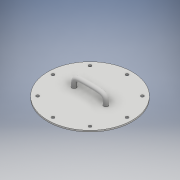
# Autodesk Inventor part: 人孔法兰
Saved by Autodesk Inventor 2018.2 (Build 222227000, 227)
## iProperties
Created: 2018-07-04
Part Number: 人孔法兰
Material: 常规
Document SubType Name: Modeling
Designer: Administrator
Density: 1 g/cm^3
Appearance: 默认
Author: Administrator
Autodesk Inventor part; units mm, degrees
ref_plane "YZ Plane" through (0, 0, 0) normal (1, 0, 0) x (0, 1, 0)
ref_plane "XZ Plane" through (0, 0, 0) normal (0, 1, 0) x (-1, 0, 0)
ref_plane "XY Plane" through (0, 0, 0) normal (0, 0, 1) x (1, 0, 0)
sketch "草图1" plane through (0, 0, 0) normal (0, 0, 1) x (1, 0, 0)
  circle A0 centre (0, 0) radius 290
  dimension "d0" = 580
  constraints: 1 centre point, 1 coincident
  measures "d0" diameter of A0
extrude "拉伸1" add sketch "草图1" along normal blind 10
sketch "草图2" plane through (0, 0, 0) normal (0, 0, 1) x (1, 0, 0)
  line L0 (0, 0) -> (255.65, 0)
  circle A0 centre (0, 0) radius 255.65
  dimension "d4" = 255.65
  constraints: 2 coincident, 2 end point, 1 horizontal, 1 horizontal alignment, 2 other
  measures "d4" distance of L0.start L0.end
hole "孔1" at (255.65, 0, 0) direction (0, 0, 1) diameter 20 end through all
pattern_circular "环形阵列1" count 8 over 360 about axis through (0, 0, -10) along (0, 0, 1) of "孔1"
sketch "草图3" plane through (0, 0, 10) normal (0, 0, 1) x (1, 0, 0)
  circle A0 centre (0, 0) radius 290 projected
  circle A1 centre (-110, 0) radius 15
  circle A2 centre (110, 0) radius 15
  dimension "d15" = 30
  dimension "d16" = 110
  dimension "d18" = 30
  dimension "d19" = 110
  constraints: 2 centre point
  measures "d15" diameter of A1
  measures "d16" distance of A0.centre A1.centre
  measures "d18" diameter of A2
  measures "d19" distance of A0.centre A2.centre
sketch "草图4" plane through (0, 0, 0) normal (0, 1, 0) x (-1, 0, 0)
  line L0 (110, 10) -> (110, 52.7861) construction
  line L1 (-110, 52.7861) -> (-110, 10) construction
  spline S0 degree 4 poles (110, 10) (110, 52.7861) (110, 76.933) (17.246, 76.933) (-17.246, 76.933) (-110, 76.933) (-110, 52.7861) (-110, 10) knots 1 1 1 1 1 1.296402 1.477939 1.714323 2 2 2 2 2
  line L2 (110, 52.7861) -> (110, 76.933) construction
  line L3 (-110, 76.933) -> (-110, 52.7861) construction
  line L4 (110, 76.933) -> (17.246, 76.933) construction
  line L5 (17.246, 76.933) -> (-17.246, 76.933) construction
  line L6 (-17.246, 76.933) -> (-110, 76.933) construction
  line L7 (0, -18.6745) -> (0, 112.0473) projected
  point P0 (0, 0)
  constraints: 3 symmetric about line, 1 vertical, 3 other
sweep "扫掠2" add profiles "草图3" path "草图4" path curves S0 contours A1
